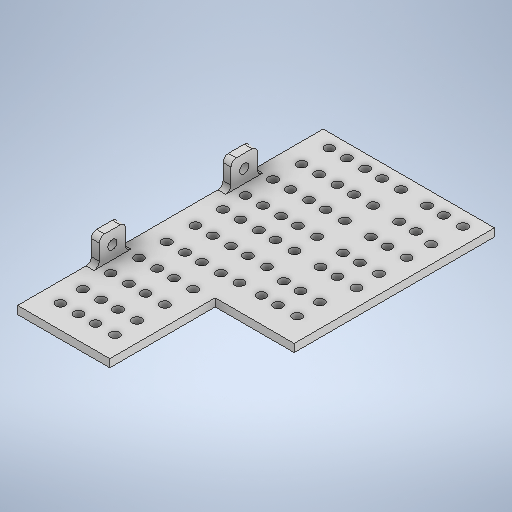
# Autodesk Inventor part: mur_étage_gauche
Saved by Autodesk Inventor 2025.1 (Build 291241000, 241)
## iProperties
Created: 2024-11-29
Part Number: mur_étage_gauche
Material: Générique
Document SubType Name: Modeling
Designer: yasmi
Density: 1 g/cm^3
Appearance: Par défaut
Author: yasmi
Autodesk Inventor part; units mm, degrees
ref_plane "YZ Plane" through (0, 0, 0) normal (1, 0, 0) x (0, 1, 0)
ref_plane "XZ Plane" through (0, 0, 0) normal (0, 1, 0) x (-1, 0, 0)
ref_plane "XY Plane" through (0, 0, 0) normal (0, 0, 1) x (1, 0, 0)
sketch "Esquisse1" plane through (0, 0, 0) normal (0, 1, 0) x (-1, 0, 0)
  line L0 (6.5, 97.6961) -> (-28.5, 97.6961)
  line L1 (6.5, -18.3039) -> (-58.5, -18.3039)
  line L2 (6.5, 97.6961) -> (6.5, -18.3039)
  line L3 (-28.5, 97.6961) -> (-28.5, 57.6961)
  line L4 (-58.5, -18.3039) -> (-58.5, 57.6961)
  line L5 (-58.5, 57.6961) -> (-28.5, 57.6961)
  circle A0 centre (-14.5383, -13.166) radius 1.75
  circle A1 centre (-20.9, -13.166) radius 1.75
  circle A2 centre (-28.1732, -13.166) radius 1.75
  circle A3 centre (-28.1732, -2.6467) radius 1.75
  circle A4 centre (-0.9853, -2.6467) radius 1.75
  circle A5 centre (-7.6096, -13.166) radius 1.75
  circle A6 centre (-7.6096, -2.6467) radius 1.75
  circle A7 centre (-20.9, -2.6467) radius 1.75
  circle A8 centre (-14.5383, -2.6467) radius 1.75
  circle A9 centre (-0.9853, -13.166) radius 1.75
  circle A10 centre (-14.1574, 7.7801) radius 1.75
  circle A11 centre (-20.5192, 7.7801) radius 1.75
  circle A12 centre (-27.7924, 7.7801) radius 1.75
  circle A13 centre (-27.7924, 18.2994) radius 1.75
  circle A14 centre (-0.6044, 18.2994) radius 1.75
  circle A15 centre (-7.2287, 7.7801) radius 1.75
  circle A16 centre (-7.2287, 18.2994) radius 1.75
  circle A17 centre (-20.5192, 18.2994) radius 1.75
  circle A18 centre (-14.1574, 18.2994) radius 1.75
  circle A19 centre (-0.6044, 7.7801) radius 1.75
  circle A20 centre (-14.5383, 27.2028) radius 1.75
  circle A21 centre (-20.9, 27.2028) radius 1.75
  circle A22 centre (-28.1732, 27.2028) radius 1.75
  circle A23 centre (-28.1732, 37.7221) radius 1.75
  circle A24 centre (-0.9853, 37.7221) radius 1.75
  circle A25 centre (-7.6096, 27.2028) radius 1.75
  circle A26 centre (-7.6096, 37.7221) radius 1.75
  circle A27 centre (-20.9, 37.7221) radius 1.75
  circle A28 centre (-14.5383, 37.7221) radius 1.75
  circle A29 centre (-0.9853, 27.2028) radius 1.75
  circle A30 centre (-14.2354, 48.5298) radius 1.75
  circle A31 centre (-7.8736, 48.5298) radius 1.75
  circle A32 centre (-0.9449, 48.5298) radius 1.75
  circle A33 centre (-21.5086, 59.0491) radius 1.75
  circle A34 centre (-14.2354, 59.0491) radius 1.75
  circle A35 centre (-7.8736, 59.0491) radius 1.75
  circle A36 centre (-0.9449, 59.0491) radius 1.75
  circle A37 centre (-21.5086, 48.5298) radius 1.75
  circle A38 centre (-13.8545, 69.4759) radius 1.75
  circle A39 centre (-7.4928, 69.4759) radius 1.75
  circle A40 centre (-0.564, 69.4759) radius 1.75
  circle A41 centre (-21.1277, 79.9952) radius 1.75
  circle A42 centre (-13.8545, 79.9952) radius 1.75
  circle A43 centre (-7.4928, 79.9952) radius 1.75
  circle A44 centre (-0.564, 79.9952) radius 1.75
  circle A45 centre (-21.1277, 69.4759) radius 1.75
  circle A46 centre (-14.2354, 88.8986) radius 1.75
  circle A47 centre (-7.8736, 88.8986) radius 1.75
  circle A48 centre (-0.9449, 88.8986) radius 1.75
  circle A49 centre (-21.6, 88.8961) radius 1.75
  circle A50 centre (-44.781, -12.7852) radius 1.75
  circle A51 centre (-38.4192, -12.7852) radius 1.75
  circle A52 centre (-51.9, -0.9374) radius 1.75
  circle A53 centre (-44.781, -2.2659) radius 1.75
  circle A54 centre (-38.4192, -2.2659) radius 1.75
  circle A55 centre (-52.0542, -12.7852) radius 1.75
  circle A56 centre (-44.4002, 8.1609) radius 1.75
  circle A57 centre (-38.0384, 8.1609) radius 1.75
  circle A58 centre (-51.6734, 18.6802) radius 1.75
  circle A59 centre (-44.4002, 18.6802) radius 1.75
  circle A60 centre (-38.0384, 18.6802) radius 1.75
  circle A61 centre (-51.6734, 8.1609) radius 1.75
  circle A62 centre (-44.781, 27.5837) radius 1.75
  circle A63 centre (-38.4192, 27.5837) radius 1.75
  circle A64 centre (-52.0542, 27.5837) radius 1.75
  circle A65 centre (-36.1026, 39.249) radius 1.75
  circle A66 centre (-49.7376, 39.249) radius 1.75
  circle A67 centre (-42.8452, 48.1525) radius 1.75
  circle A68 centre (-50.1185, 48.1525) radius 1.75
  circle A69 centre (-42.4644, 39.249) radius 1.75
  circle A70 centre (-36.4835, 48.1525) radius 1.75
  circle A71 centre (-28.1732, 48.1525) radius 1.75
  line L6 (3.5, 9.6961) -> (6.5, 9.6961)
  line L7 (6.5, 9.6961) -> (6.5, 19.6961)
  line L8 (6.5, 19.6961) -> (3.5, 19.6961)
  line L9 (3.5, 19.6961) -> (3.5, 9.6961)
  line L10 (3.5, 9.6961) -> (6.5, 19.6961) construction
  line L11 (6.5, 9.6961) -> (3.5, 19.6961) construction
  line L12 (3.5, 59.6961) -> (6.5, 59.6961)
  line L13 (6.5, 59.6961) -> (6.5, 69.6961)
  line L14 (6.5, 69.6961) -> (3.5, 69.6961)
  line L15 (3.5, 69.6961) -> (3.5, 59.6961)
  line L16 (3.5, 59.6961) -> (6.5, 69.6961) construction
  line L17 (6.5, 59.6961) -> (3.5, 69.6961) construction
  point P0 (0, 0)
  point P1 (-47.865, 53.9077)
  point P2 (5, 14.6961)
  point P3 (5, 64.6961)
  dimension "d0" = 35
  dimension "d1" = 65
  dimension "d2" = 116
  dimension "d3" = 40
  dimension "d4" = 76
  dimension "d10" = 17.3665
  dimension "d11" = 6.6
  dimension "d30" = 1.5
  dimension "d31" = 1.5
  dimension "d32" = 33
  dimension "d33" = 33
  dimension "d34" = 3
  dimension "d35" = 3
  dimension "d36" = 10
  dimension "d37" = 10
  dimension "d51" = 6.9
  dimension "d52" = 8.8
  constraints: 72 centre point, 36 end point, 4 horizontal, 4 midpoint, 4 parallel, 3 perpendicular, 2 vertical
  measures "d0" distance of L0.start L0.end
  measures "d1" distance of L1.start L1.end
  measures "d2" distance of L0.start L1.start
  measures "d3" distance of L0.end L3.end
  measures "d4" distance of L1.end L4.end
  measures "d10" distance from line of L1 A52.centre
  measures "d11" distance from line of A52.centre L4
  measures "d30" distance from line of L2 point (5, 14.696)
  measures "d31" distance from line of L2 point (5, 64.696)
  measures "d32" distance from line of L1 point (5, 14.696)
  measures "d33" distance from line of L0 point (5, 64.696)
  measures "d34" distance of L8.end L7.end
  measures "d35" distance of L14.end L13.end
  measures "d36" distance of L13.end L12.end
  measures "d37" distance of L8.end L6.start
  measures "d51" distance from line of L3 A49.centre
  measures "d52" distance from line of L0 A49.centre
extrude "Extrusion6" add sketch "Esquisse1" along normal blind 3 contours L2 L14 L15 L12 L8 L9 L6 L1 L4 L5 L3 L0
extrude "Extrusion7" add sketch "Esquisse1" along normal blind 13 contours L2 L6 L9 L8
extrude "Extrusion8" add sketch "Esquisse1" along normal blind 13 contours L2 L12 L15 L14
sketch "Esquisse6" plane through (-3.5, 3, 9.6961) normal (1, 0, 0) x (0, 0, -1)
  line L0 (0, 0) -> (0, 10) projected
  line L1 (-10, 0) -> (-10, 10) projected
  line L2 (0, 0) -> (-10, 10)
  line L3 (-10, 10) -> (0, 10)
  line L4 (0, 10) -> (-10, 0)
  circle A0 centre (-5, 5) radius 1.75
  line L5 (-50, 0) -> (-50, 10) projected
  line L6 (-50, 0) -> (-60, 10)
  line L7 (-60, 10) -> (-50, 10)
  line L8 (-60, 0) -> (-60, 10) projected
  line L9 (-50, 10) -> (-60, 0)
  circle A1 centre (-55, 5) radius 1.75
  line L10 (-48, 0) -> (28, 0) projected
  line L11 (-88, 0) -> (-48, 0) projected
  point P0 (9.6961, -3)
  point P1 (-5, 5)
  point P2 (-55, 5)
  dimension "d44" = 3.5
  dimension "d45" = 3.5
  dimension "d46" = 5
  dimension "d47" = 5
  constraints: 12 end point, 4 midpoint, 4 perpendicular, 2 centre point, 1 coincident
  measures "d44" diameter of A0
  measures "d45" diameter of A1
  measures "d46" distance from line of L10 point (-5, 5)
  measures "d47" distance from line of L11 point (-55, 5)
extrude "Extrusion9" cut sketch "Esquisse6" against normal blind 3 contours A0 L4 L2 | L2 L4 A0 | L4 L2 A0 | L4 A0 L2 | A1 L9 L6 | L6 L9 A1 | L9 L6 A1 | L9 A1 L6
fillet "Congé2" radius 2 8 edges at (-5, 13, 69.6961) (-5, 3, 69.6961) (-5, 13, 59.6961) (-5, 3, 19.6961) (-5, 13, 19.6961) (-5, 13, 9.6961) (-5, 3, 9.6961) (-5, 3, 59.6961)
